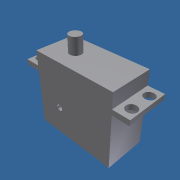
# Autodesk Inventor part: ServoFutabaS3003
Saved by Autodesk Inventor 2012 (Build 160160000, 160)
## iProperties
Created: 2014-03-29
Part Number: ServoFutabaS3003
Material: Default
Document SubType Name: Modeling
Designer: Admin
Density: 1 g/cm^3
Author: Admin
Autodesk Inventor part; units mm, degrees
ref_plane "YZ Plane" through (0, 0, 0) normal (1, 0, 0) x (0, 1, 0)
ref_plane "XZ Plane" through (0, 0, 0) normal (0, 1, 0) x (-1, 0, 0)
ref_plane "XY Plane" through (0, 0, 0) normal (0, 0, 1) x (1, 0, 0)
sketch "Sketch1" plane through (0, 0, 0) normal (0, 0, 1) x (1, 0, 0)
  line L0 (-28.21, 0) -> (28.21, 0) projected
  line L1 (0, -13.86) -> (0, 13.86) projected
  line L2 (-20.15, 9.9) -> (20.15, 9.9)
  line L3 (20.15, 9.9) -> (20.15, -9.9)
  line L4 (20.15, -9.9) -> (-20.15, -9.9)
  line L5 (-20.15, -9.9) -> (-20.15, 9.9)
  point P0 (0, 0)
  dimension "d0" = 19.8
  dimension "d1" = 9.9
  dimension "d2" = 40.3
  dimension "d3" = 20.15
  constraints: 8 end point, 2 parallel, 1 horizontal, 1 perpendicular
  measures "d0" distance of L4.end L2.start
  measures "d1" distance between parallel lines of L0 L2
  measures "d2" distance of L2.start L2.end
  measures "d3" distance between parallel lines of L1 L5
extrude "Extrusion1" add sketch "Sketch1" along normal blind 26.6
sketch "Sketch2" plane through (0, 0, 26.6) normal (0, 0, 1) x (1, 0, 0)
  line L0 (-27.75, 9.9) -> (27.75, 9.9)
  line L1 (27.75, 9.9) -> (27.75, -9.9)
  line L2 (27.75, -9.9) -> (-27.75, -9.9)
  line L3 (-27.75, -9.9) -> (-27.75, 9.9)
  line L4 (-38.85, 0) -> (38.85, 0) projected
  line L5 (0, -13.86) -> (0, 13.86) projected
  point P0 (0, 0)
  dimension "d6" = 55.5
  dimension "d7" = 19.8
  dimension "d8" = 27.75
  dimension "d9" = 9.9
  constraints: 8 end point, 2 parallel, 1 horizontal, 1 perpendicular
  measures "d6" distance of L1.end L2.end
  measures "d7" distance of L0.end L1.end
  measures "d8" distance between parallel lines of L5 L1
  measures "d9" distance between parallel lines of L4 L0
extrude "Extrusion2" add sketch "Sketch2" along normal blind 2.55
sketch "Sketch3" plane through (0, 0, 29.15) normal (0, 0, 1) x (1, 0, 0)
  line L0 (-27.75, 9.9) -> (27.75, 9.9) projected
  circle A0 centre (-24.5, 5) radius 2.5
  circle A1 centre (-24.5, -5) radius 2.5
  circle A2 centre (24.5, 5) radius 2.5
  circle A3 centre (24.5, -5) radius 2.5
  point P0 (-27.75, -9.9)
  point P1 (0, 0)
  dimension "d12" = 5
  dimension "d13" = 5
  dimension "d14" = 5
  dimension "d15" = 5
  dimension "d16" = 10
  dimension "d17" = 10
  dimension "d18" = 4.9
  dimension "d19" = 19.8
  dimension "d20" = 4.9
  dimension "d21" = 49
  dimension "d22" = 24.5
  constraints: 4 centre point
  measures "d12" diameter of A0
  measures "d13" diameter of A1
  measures "d14" diameter of A2
  measures "d15" diameter of A3
  measures "d16" distance of A0.centre A1.centre
  measures "d17" distance of A2.centre A3.centre
  measures "d18" distance from line of L0 A0.centre
  measures "d19" distance of point (-27.75, -9.9) L0.start
  measures "d20" distance from line of L0 A2.centre
  measures "d21" distance of A2.centre A0.centre
  measures "d22" horizontal distance of point (0, 0) A0.centre
extrude "Extrusion3" cut sketch "Sketch3" against normal blind 2.55
sketch "Sketch4" plane through (0, 0, 29.15) normal (0, 0, 1) x (1, 0, 0)
  line L0 (-27.75, 9.9) -> (27.75, 9.9) projected
  line L1 (27.75, -9.9) -> (-27.75, -9.9) projected
  line L2 (-20.15, -9.9) -> (-20.15, 9.9) projected
  line L3 (20.15, 9.9) -> (20.15, -9.9) projected
  point P0 (0, 0)
extrude "Extrusion4" add sketch "Sketch4" along normal blind 7
sketch "Sketch5" plane through (0, 0, 36.15) normal (0, 0, 1) x (1, 0, 0)
  circle A0 centre (-7.9, 0) radius 3
  line L0 (-27.75, -9.9) -> (-27.75, 9.9) projected
  point P0 (0, 0)
  dimension "d27" = 6
  dimension "d28" = 19.85
  constraints: 1 centre point
  measures "d27" diameter of A0
  measures "d28" distance from line of L0 A0.centre
extrude "Extrusion5" add sketch "Sketch5" along normal blind 7.85
sketch "Sketch6" plane through (0, 0, 0) normal (0, 0, -1) x (-1, 0, 0)
  line L0 (20.15, -9.9) -> (20.15, 9.9) projected
  line L1 (20.15, 2.5) -> (26.15, 2.5)
  line L2 (26.15, 2.5) -> (26.15, -2.5)
  line L3 (26.15, -2.5) -> (20.15, -2.5)
  line L4 (20.15, -2.5) -> (20.15, 2.5)
  point P0 (0, 0)
  dimension "d31" = 6
  dimension "d32" = 2.5
  dimension "d33" = 5
  constraints: 8 end point, 2 parallel, 1 horizontal, 1 perpendicular, 1 point on line
  measures "d31" distance of L2.end L3.end
  measures "d32" distance from line of point (0, 0) L1
  measures "d33" distance of L1.end L2.end
extrude "Extrusion6" add sketch "Sketch6" against normal blind 5
sketch "Sketch7" plane through (-20.15, -9.9, 0) normal (0, -1, 0) x (1, 0, 0)
  line L0 (40.3, 0) -> (0, 0) projected
  line L1 (9.25, 44) -> (15.25, 44)
  line L2 (9.25, 36.15) -> (9.25, 44) projected
  line L3 (15.25, 36.15) -> (15.25, 44) projected
  circle A0 centre (12.25, 14) radius 1.5
  point P0 (20.15, 0)
  dimension "d36" = 3
  dimension "d37" = 30
  constraints: 2 end point, 1 centre point, 1 horizontal, 2 other
  measures "d36" diameter of A0
  measures "d37" distance from line of A0.centre L1
extrude "Extrusion7" cut sketch "Sketch7" against normal through all
equation "\"d1\" = 0.5 * d0"
equation "\"d3\" = 0.5 * d2"
equation "\"d8\" = 0.5 * d6"
equation "\"d9\" = 0.5 * d7"
equation "\"d20\" = d18"
equation "\"d22\" = 0.5 * d21"
equation "\"d32\" = 0.5 * d33"
body "Solid1"
